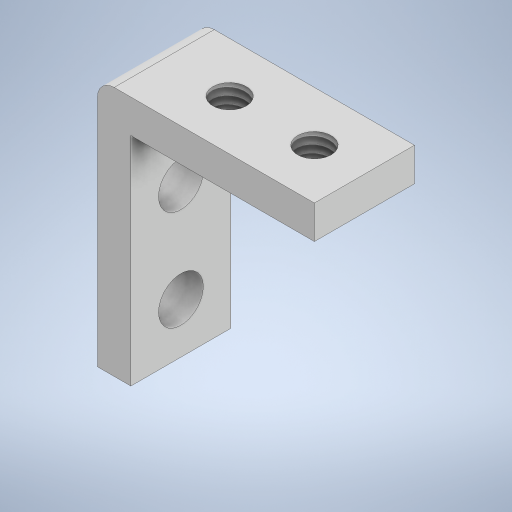
# Autodesk Inventor part: bracket
Saved by Autodesk Inventor 2024 (Build 280153000, 153)
## iProperties
Created: 2023-10-02
Part Number: bracket
Material: Generic
Document SubType Name: Modeling
Designer: Alexander Pollak
Density: 1 g/cm^3
Appearance: Default
Author: Alexander Pollak
Autodesk Inventor part; units mm, degrees
ref_plane "YZ Plane" through (0, 0, 0) normal (1, 0, 0) x (0, 1, 0)
ref_plane "XZ Plane" through (0, 0, 0) normal (0, 1, 0) x (-1, 0, 0)
ref_plane "XY Plane" through (0, 0, 0) normal (0, 0, 1) x (1, 0, 0)
sketch "Sketch1" plane through (0, 0, 0) normal (1, 0, 0) x (0, 1, 0)
  line L0 (-7.5, 3) -> (7.5, 3)
  line L1 (7.5, 3) -> (7.5, -3)
  line L2 (7.5, -3) -> (-7.5, -3)
  line L3 (-7.5, -3) -> (-7.5, 3)
  line L4 (-7.5, 3) -> (7.5, -3) construction
  line L5 (7.5, 3) -> (-7.5, -3) construction
  point P0 (0, 0)
  dimension "d0" = 15
  dimension "d1" = 6
  constraints: 12 end point, 2 midpoint, 2 parallel, 1 horizontal, 1 perpendicular
  measures "d0" distance of L1.end L2.end
  measures "d1" distance of L0.end L1.end
extrude "Extrusion1" add sketch "Sketch1" along normal blind 2
sketch "Sketch2" plane through (2, 0, 0) normal (1, 0, 0) x (0, 0, -1)
  line L0 (3, 7.5) -> (-3, 7.5) projected
  line L1 (3, -7.5) -> (3, 7.5) projected
  line L2 (-3, 7.5) -> (3, 7.5)
  line L3 (3, 7.5) -> (3, 5.5)
  line L4 (3, 5.5) -> (-3, 5.5)
  line L5 (-3, 5.5) -> (-3, 7.5)
  point P0 (0, 0)
  dimension "d4" = 2
  constraints: 8 end point, 2 parallel, 1 horizontal, 1 perpendicular, 1 point on line
  measures "d4" distance of L2.end L3.end
extrude "Extrusion2" add sketch "Sketch2" along normal blind 11
fillet "Fillet1" radius 1 1 edges at (0, 7.5, 0)
sketch "Sketch3" plane through (13, 7.5, 3) normal (0, 1, 0) x (1, 0, 0)
  line L0 (0, 6) -> (0, 0) construction
  line L1 (0, 3) -> (-12, 3) construction
  line L2 (-12, 0) -> (-12, 6) construction
  point P0 (-13, 3)
  point P1 (-8.08, 3)
  point P2 (-3, 3)
  dimension "d8" = 5.08
  dimension "d9" = 3
  constraints: 3 midpoint, 2 end point, 2 point on line
  measures "d8" distance of point (-3, 3) point (-8.08, 3)
  measures "d9" distance of point (0, 3) point (-3, 3)
hole "Hole1" at (4.92, 7.5, 0) at (10, 7.5, 0) direction (0, -1, 0) diameter 2.013 end through all thread size "M2.5x0.45" class "6H" standard "ISO Metric profile"
sketch "Sketch4" plane through (2, 0, 0) normal (1, 0, 0) x (0, 0, -1)
  line L0 (-3, -7.5) -> (3, -7.5) construction
  line L1 (0, -7.5) -> (0, 5.5) construction
  line L2 (-3, 5.5) -> (3, 5.5) construction
  line L3 (3, 7.5) -> (-3, 7.5) construction
  point P0 (0, 0)
  point P1 (0, 1.5)
  point P2 (0, -4.5)
  dimension "d17" = 6
  dimension "d18" = 6
  constraints: 2 end point, 2 midpoint, 2 point on line
  measures "d17" distance of point (0, -4.5) point (0, 1.5)
  measures "d18" distance from line of L3 point (0, 1.5)
hole "Hole2" at (2, 1.5, 0) at (2, -4.5, 0) direction (-1, 0, 0) diameter 2.69 end through all
body "Solid1"
